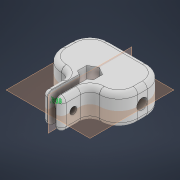
# Autodesk Inventor part: Bad Intake Bracket v2
Saved by Autodesk Inventor 2022 (Build 260153000, 153)
## iProperties
Created: 2022-02-03
Part Number: Bad Intake Bracket v2
Material: Generic
Document SubType Name: Modeling
Designer: izack
Density: 1 g/cm^3
Appearance: Default
Author: izack
Autodesk Inventor part; units mm, degrees
ref_plane "YZ Plane" through (0, 0, 0) normal (1, 0, 0) x (0, 1, 0)
ref_plane "XZ Plane" through (0, 0, 0) normal (0, 1, 0) x (-1, 0, 0)
ref_plane "XY Plane" through (0, 0, 0) normal (0, 0, 1) x (1, 0, 0)
sketch "Sketch1" plane through (0, 0, 0) normal (0, 1, 0) x (-1, 0, 0)
  circle A0 centre (0, 0) radius 2.65
  line L0 (2.65, -1.53) -> (0, -3.06)
  line L1 (0, -3.06) -> (-2.65, -1.53)
  line L2 (-2.65, -1.53) -> (-2.65, 1.53)
  line L3 (-2.65, 1.53) -> (0, 3.06)
  line L4 (0, 3.06) -> (2.65, 1.53)
  line L5 (2.65, 1.53) -> (2.65, -1.53)
  line L6 (1.325, 12.7) -> (-1.325, 12.7)
  line L7 (-12.7, -3.2069) -> (-12.7, -6.35)
  line L8 (-6.35, -12.7) -> (6.35, -12.7)
  line L9 (12.7, -6.35) -> (12.7, -3.2069)
  line L10 (12.7, 12.7) -> (-12.7, -12.7) construction
  line L11 (-12.7, 12.7) -> (12.7, -12.7) construction
  arc A1 (-12.7, -6.35) -> (-6.35, -12.7) centre (-6.35, -6.35) ccw
  arc A2 (6.35, -12.7) -> (12.7, -6.35) centre (6.35, -6.35) ccw
  line L12 (1.325, 2.295) -> (1.325, 12.7)
  line L13 (-1.325, 2.295) -> (-1.325, 12.7)
  circle A3 centre (0, 0) radius 4.445
  line L14 (6.3181, 3.1431) -> (6.35, 3.1431)
  line L15 (-6.3181, 3.1431) -> (-6.35, 3.1431)
  arc A4 (-6.35, 3.1431) -> (-12.7, -3.2069) centre (-6.35, -3.2069) ccw
  arc A5 (12.7, -3.2069) -> (6.35, 3.1431) centre (6.35, -3.2069) ccw
  line L16 (-3.1431, 6.3181) -> (-3.1431, 11.1252)
  line L17 (-1.5683, 12.7) -> (-1.325, 12.7)
  line L18 (1.325, 12.7) -> (1.5683, 12.7)
  line L19 (3.1431, 11.1252) -> (3.1431, 6.3181)
  arc A6 (-6.3181, 3.1431) -> (-3.1431, 6.3181) centre (-6.3181, 6.3181) ccw
  arc A7 (3.1431, 6.3181) -> (6.3181, 3.1431) centre (6.3181, 6.3181) ccw
  arc A8 (3.1431, 11.1252) -> (1.5683, 12.7) centre (1.5683, 11.1252) ccw
  arc A9 (-1.5683, 12.7) -> (-3.1431, 11.1252) centre (-1.5683, 11.1252) ccw
  point P0 (2.65, 0)
  point P1 (3.1431, 3.1431)
  point P2 (-3.1431, 3.1431)
  point P3 (-12.7, 3.1431)
  point P4 (3.1431, 12.7)
  dimension "d0" = 5.3
  dimension "d1" = 25.4
  dimension "d2" = 25.4
  dimension "d4" = 8.89
  dimension "d5" = 6.35
  dimension "d6" = 3.175
  dimension "d7" = 1.5748
  constraints: 40 end point, 20 point on line, 18 point on circle, 16 tangent, 9 centre point, 6 perpendicular, 5 midpoint, 3 coincident, 3 equal radius, 3 parallel, 1 horizontal, 1 horizontal alignment, 15 other
  measures "d1" distance of L11.end L10.end
  measures "d2" distance of L10.end L11.start
  measures "d4" diameter of A3
  measures "d5" radius of A4
  measures "d6" radius of A6
  measures "d7" radius of A8
extrude "Extrusion1" add sketch "Sketch1" along normal blind 10 contours L5 L4 L12 A3 L13 L3 L2 L1 L0 | L12 L18 A8 L19 A7 L14 A5 L9 A2 L8 A1 L7 A4 L15 A6 L16 A9 L17 L13 A3
fillet "Fillet1" radius 1.5875 34 edges at (-10.8401, 10, 1.2832) (-6.334, 10, 3.1431) (-4.073, 10, 4.073) (-3.1431, 10, 8.7216) (-2.6818, 10, 12.2388) (-1.4466, 10, 12.7) (-10.8401, 10, -10.8401) (0, 10, -12.7) (10.8401, 10, -10.8401) (12.7, 10, -4.7785) (10.8401, 10, 1.2832) (6.334, 10, 3.1431) (4.073, 10, 4.073) (3.1431, 10, 8.7216) (2.6818, 10, 12.2388) (1.4466, 10, 12.7) (-12.7, 10, -4.7785) (-10.8401, 0, 1.2832) (-6.334, 0, 3.1431) (-4.073, 0, 4.073) (-3.1431, 0, 8.7216) (-2.6818, 0, 12.2388) (-1.4466, 0, 12.7) (-10.8401, 0, -10.8401) (0, 0, -12.7) (10.8401, 0, -10.8401) (12.7, 0, -4.7785) (10.8401, 0, 1.2832) (6.334, 0, 3.1431) (4.073, 0, 4.073) (3.1431, 0, 8.7216) (2.6818, 0, 12.2388) (1.4466, 0, 12.7) (-12.7, 0, -4.7785)
sketch "Sketch2" plane through (-3.1431, 1.5875, 11.1252) normal (-1, 0, 0) x (0, 0, 1)
  line L0 (-4.8071, 0) -> (-4.8071, 6.825) construction
  line L1 (-4.8071, 3.4125) -> (0, 3.4125) construction
  line L2 (0, 0) -> (0, 6.825) construction
  line L3 (-4.8071, 0) -> (0, 0) construction
  line L4 (-2.4036, 0) -> (-2.4036, 6.825) construction
  line L5 (-4.8071, 6.825) -> (0, 6.825) construction
  circle A0 centre (-2.4036, 3.4125) radius 1.15
  circle A1 centre (-2.4036, 3.4125) radius 1.75
  point P0 (-11.1252, -1.5875)
  dimension "d11" = 2.3
  dimension "d12" = 3.5
  constraints: 5 midpoint, 4 end point, 2 centre point, 1 coincident
  measures "d11" diameter of A0
  measures "d12" diameter of A1
extrude "Extrusion2" cut sketch "Sketch2" against normal up to surface (1.8181 mm away) contours A0 | A1
extrude "Extrusion3" cut sketch "Sketch2" against normal up to surface (6.2862 mm away) contours A0
ref_plane "Work Plane1" through (0, 5, 0) normal (0, 1, 0) x (1, 0, 0)
sketch "Sketch3" plane through (0, 5, 0) normal (0, 1, 0) x (1, 0, 0)
  line L0 (-12.7508, 4.6668) -> (-6.1607, 4.6668)
  line L1 (-5.0471, 5.128) -> (-2.6519, 7.5232)
  line L2 (0, 13.8984) -> (0, -13.9494) construction
  line L3 (12.7508, 4.6668) -> (6.1607, 4.6668)
  line L4 (5.0471, 5.128) -> (2.6519, 7.5232)
  arc A0 (5.0471, 5.128) -> (6.1607, 4.6668) centre (6.1607, 6.2416) ccw
  arc A1 (-6.1607, 4.6668) -> (-5.0471, 5.128) centre (-6.1607, 6.2416) ccw
  point P0 (0, 0)
  point P1 (-5.5084, 4.6668)
  point P2 (5.5084, 4.6668)
  dimension "d17" = 135
  dimension "d18" = 1.5748
  constraints: 10 end point, 4 point on circle, 4 point on line, 4 tangent, 3 symmetric about line, 2 centre point, 1 equal radius, 1 horizontal, 1 vertical
  measures "d17" angle of L1 L0
  measures "d18" radius of A0
sketch "Sketch4" plane through (12.7, 1.5875, -6.35) normal (1, 0, 0) x (0, 0, -1)
  circle A0 centre (-1.6832, 3.4125) radius 1.27
  line L0 (7.5484, 3.4125) -> (-20.2994, 3.4125) construction
  point P0 (-6.35, -1.5875)
  dimension "d19" = 2.54
  constraints: 1 centre point, 1 coincident
  measures "d19" diameter of A0
sweep "Sweep1" cut profiles "Sketch4" path "Sketch3" path curves L3 A0 L4
ref_plane "Work Plane2" through (0, 1.5875, -6.35) normal (1, 0, 0) x (0, 0, -1)
chamfer "Chamfer1" distance 0.508 distance2 3.175 1 edges at (12.7, 5, -3.3968) measured on face at (12.7, 5, -3.2968)
mirror "Mirror1" about plane through (0, 1.5875, -6.35) normal (1, 0, 0) of "Sweep1"
chamfer "Chamfer2" distance 0.508 distance2 3.175 1 edges at (-12.7, 5, -3.3968) measured on face at (-12.7, 5, -3.2968)
body "Solid1"
